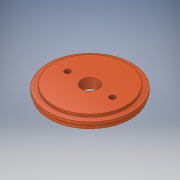
# Autodesk Inventor part: upper_thermal_barrier
Saved by Autodesk Inventor 2017 SP1 (Build 210196100, 196)
## iProperties
Created: 2016-10-21
Part Number: upper_thermal_barrier
Material: Phenolic Resin
Document SubType Name: Modeling
Designer: cflannery
Density: 1.38 g/cm^3
Appearance: Smooth - Light Orange
Author: cflannery
Autodesk Inventor part; units mm, degrees
ref_plane "YZ Plane" through (0, 0, 0) normal (1, 0, 0) x (0, 1, 0)
ref_plane "XZ Plane" through (0, 0, 0) normal (0, 1, 0) x (-1, 0, 0)
ref_plane "XY Plane" through (0, 0, 0) normal (0, 0, 1) x (1, 0, 0)
sketch "Sketch1" plane through (0, 0, 0) normal (0, 1, 0) x (-1, 0, 0)
  circle A0 centre (0, 0) radius 92.075
  dimension "d0" = 184.15
  constraints: 1 centre point, 1 coincident
  measures "d0" diameter of A0
extrude "Extrusion1" add sketch "Sketch1" along normal blind 6.35
sketch "Sketch2" plane through (0, 6.35, 0) normal (0, 1, 0) x (1, 0, 0)
  circle A0 centre (0, 0) radius 88.9
  dimension "d3" = 177.8
  constraints: 1 centre point, 1 coincident
  measures "d3" diameter of A0
extrude "Extrusion2" add sketch "Sketch2" along normal blind 3.175
sketch "Sketch3" plane through (0, 9.525, 0) normal (0, 1, 0) x (1, 0, 0)
  circle A0 centre (0, 0) radius 95.25
  dimension "d6" = 190.5
  constraints: 1 centre point, 1 coincident
  measures "d6" diameter of A0
extrude "Extrusion3" add sketch "Sketch3" along normal blind 6.35
sketch "Sketch6" plane through (0, 15.875, 0) normal (0, 1, 0) x (1, 0, 0)
  circle A0 centre (0, 0) radius 82.55
  dimension "d23" = 165.1
  constraints: 1 centre point, 1 coincident
  measures "d23" diameter of A0
extrude "Extrusion7" add sketch "Sketch6" along normal blind 6.35
sketch "Sketch7" plane through (0, 22.225, 0) normal (0, 1, 0) x (1, 0, 0)
  circle A0 centre (0, 0) radius 19.05
  circle A1 centre (-50.8, 0) radius 6.35
  circle A2 centre (50.8, 0) radius 6.35
  dimension "d27" = 38.1
  dimension "d28" = 50.8
  dimension "d29" = 50.8
  dimension "d30" = 12.7
  constraints: 3 centre point, 2 horizontal alignment, 1 coincident, 1 equal radius
  measures "d27" diameter of A0
  measures "d28" distance of point (0, 0) A1.centre
  measures "d29" distance of point (0, 0) A2.centre
  measures "d30" diameter of A1
extrude "Extrusion8" cut sketch "Sketch7" against normal through all
equation "\"d29\" = d28"
body "Solid1"
